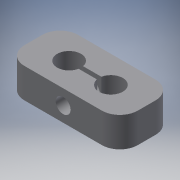
# Autodesk Inventor part: crank web2
Saved by Autodesk Inventor 2017 SP1 (Build 210196100, 196)
## iProperties
Created: 2017-06-14
Part Number: crank web2
Material: Generic
Document SubType Name: Modeling
Designer: RMcComber
Density: 1 g/cm^3
Appearance: Default
Author: RMcComber
Autodesk Inventor part; units mm, degrees
ref_plane "YZ Plane" through (0, 0, 0) normal (1, 0, 0) x (0, 1, 0)
ref_plane "XZ Plane" through (0, 0, 0) normal (0, 1, 0) x (-1, 0, 0)
ref_plane "XY Plane" through (0, 0, 0) normal (0, 0, 1) x (1, 0, 0)
sketch "Sketch1" plane through (0, 0, 0) normal (0, 0, 1) x (1, 0, 0)
  line L0 (0, 0) -> (-14, 0) construction
  circle A0 centre (-14, 0) radius 4
  circle A1 centre (0, 0) radius 4
  line L1 (12, -9) -> (-26, -9)
  line L2 (-26, -9) -> (-26, 9)
  line L3 (-26, 9) -> (12, 9)
  line L4 (12, 9) -> (12, -9)
  line L5 (12, -9) -> (-26, 9) construction
  line L6 (-26, -9) -> (12, 9) construction
  point P0 (-7, 0)
  dimension "d0" = 8
  dimension "d1" = 14
  dimension "d2" = 12
  dimension "d3" = 18
  dimension "d13" = 38
  constraints: 14 end point, 3 midpoint, 2 centre point, 2 coincident, 2 horizontal, 2 parallel, 1 equal radius, 1 perpendicular
  measures "d0" diameter of A0
  measures "d1" distance of L0.start L0.end
  measures "d2" distance from line of L0.end L2
  measures "d3" distance of L3.end L1.start
  measures "d13" distance of L1.start L1.end
extrude "Extrusion1" add sketch "Sketch1" along normal blind 10
sketch "Sketch2" plane through (-26, 9, 0) normal (0, 1, 0) x (1, 0, 0)
  circle A0 centre (19, -5) radius 2.5
  line L0 (19, -5) -> (0, -5) construction
  line L1 (0, 0) -> (0, -10) construction
  point P0 (26, 0)
  dimension "d6" = 5
  dimension "d17" = 19
  constraints: 2 end point, 1 centre point, 1 midpoint
  measures "d6" diameter of A0
  measures "d17" distance of L0.start L0.end
extrude "Extrusion2" cut sketch "Sketch2" against normal through all
fillet "Fillet1" radius 6 4 edges at (12, 9, 5) (-26, 9, 5) (-26, -9, 5) (12, -9, 5)
sketch "Sketch3" plane through (0, 0, 10) normal (0, 0, 1) x (1, 0, 0)
  line L0 (-20, -9) -> (6, -9) projected
  circle A0 centre (0, 0) radius 4 projected
  circle A1 centre (-14, 0) radius 4 projected
  line L1 (-14, 0) -> (0, 0) construction
  line L2 (0, -0.75) -> (-14, -0.75)
  line L3 (-14, -0.75) -> (-14, 0.75)
  line L4 (-14, 0.75) -> (0, 0.75)
  line L5 (0, 0.75) -> (0, -0.75)
  line L6 (0, -0.75) -> (-14, 0.75) construction
  line L7 (-14, -0.75) -> (0, 0.75) construction
  point P0 (-7, 0)
  dimension "d10" = 1.5
  constraints: 14 end point, 4 midpoint, 3 parallel, 1 horizontal, 1 perpendicular
  measures "d10" distance of L2.end L3.end
extrude "Extrusion3" cut sketch "Sketch3" against normal through all contours L4 L5 L2 A0 | A0 L2 A1 L4 | A1 L2 L3 L4 picked at (-1.3307, -0.0838) picked at (-12.6667, 0)
sketch "Sketch4" plane through (0, 0, 10) normal (0, 0, 1) x (1, 0, 0)
  line L0 (-10.0709, 0.75) -> (-3.9291, 0.75) construction
  arc A0 (-3.9291, -0.75) -> (-3.9291, 0.75) centre (0, 0) ccw construction
  line L1 (-3.9291, -0.75) -> (-10.0709, -0.75) construction
  arc A1 (-10.0709, 0.75) -> (-10.0709, -0.75) centre (-14, 0) ccw construction
  arc A2 (6, -9) -> (12, -3) centre (6, -3) ccw construction
  line L2 (12, -3) -> (12, 3) construction
  arc A3 (12, 3) -> (6, 9) centre (6, 3) ccw construction
  line L3 (6, 9) -> (-20, 9) construction
  arc A4 (-20, 9) -> (-26, 3) centre (-20, 3) ccw construction
  line L4 (-26, 3) -> (-26, -3) construction
  arc A5 (-26, -3) -> (-20, -9) centre (-20, -3) ccw construction
  line L5 (-20, -9) -> (6, -9) construction
  line L6 (-9.2375, -4.7625) -> (-18.7625, -4.7625)
  line L7 (-18.7625, -4.7625) -> (-18.7625, 4.7625)
  line L8 (-18.7625, 4.7625) -> (-9.2375, 4.7625)
  line L9 (-9.2375, 4.7625) -> (-9.2375, -4.7625)
  line L10 (-9.2375, -4.7625) -> (-18.7625, 4.7625) construction
  line L11 (-18.7625, -4.7625) -> (-9.2375, 4.7625) construction
  dimension "d14" = 9.525
  constraints: 12 end point, 2 midpoint, 2 parallel, 2 perpendicular, 1 horizontal
  measures "d14" distance of L7.end L8.end
extrude "Extrusion4" [suppressed]
body "Solid1"
